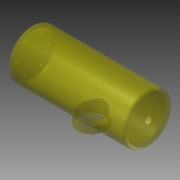
# Autodesk Inventor part: X-Ray Tube
Saved by Autodesk Inventor 2015 (Build 190159000, 159)
## iProperties
Created: 2015-03-02
Part Number: X-Ray Tube
Material: Glass
Document SubType Name: Modeling
Designer: pltwe4
Density: 2.18 g/cm^3
Appearance: Clear - Yellow
Author: pltwe4
Autodesk Inventor part; units mm, degrees
ref_plane "XZ Plane" through (0, 0, 0) normal (0, 1, 0) x (-1, 0, 0)
ref_plane "XY Plane" through (0, 0, 0) normal (0, 0, 1) x (1, 0, 0)
sketch "Sketch1" plane through (0, 0, 0) normal (0, 0, 1) x (1, 0, 0)
  circle A0 centre (0, 0) radius 14.925
  dimension "d0" = 29.85
  constraints: 1 centre point, 1 coincident
  measures "d0" diameter of A0
extrude "Extrusion1" add sketch "Sketch1" along normal mid plane 71.7
ref_plane "Work Plane1" through (14.925, 0, 0) normal (1, 0, 0) x (0, 1, 0)
sketch "Sketch2" plane through (14.925, 0, 0) normal (1, 0, 0) x (0, 1, 0)
  line L0 (-14.925, -35.85) -> (14.925, -35.85) projected
  line L1 (14.925, 35.85) -> (-14.925, 35.85) projected
  circle A0 centre (0, -1.03) radius 8.575
  line L2 (0, 50.19) -> (0, -50.19) projected
  circle A1 centre (0, -1.03) radius 7.575
  point P0 (0, 0)
  dimension "d3" = 34.82
  dimension "d4" = 17.15
  dimension "d49" = 1
  constraints: 2 centre point, 1 coincident, 1 point on line
  measures "d3" distance from line of L0 A0.centre
  measures "d4" diameter of A0
  measures "d49" radial gap between concentric circles of A1 A0
extrude "Extrusion2" add sketch "Sketch2" against normal up to surface round surface about axis through (0, 0, 0) along (0, 0, 1) radius 14.925 far side no
sketch "Sketch9" plane through (0, 0, 35.85) normal (0, 0, 1) x (1, 0, 0)
  point P0 (0, 0)
sketch "Sketch10" plane through (0, 0, 35.85) normal (0, 0, 1) x (1, 0, 0)
  circle A0 centre (0, 0) radius 12.925
  circle A1 centre (0, 0) radius 14.925 projected
  dimension "d31" = 2
  constraints: 1 centre point, 1 coincident
  measures "d31" radial gap between concentric circles of A1 A0
extrude "Extrusion11" cut sketch "Sketch10" against normal blind 70.7 contours A0
fillet "Fillet3" radius 2 1 edges at (-12.925, 0, -34.85)
fillet "Fillet4" radius 2 1 edges at (-14.925, 0, -35.85)
sketch "Sketch11" plane through (0, 0, 35.85) normal (0, 0, 1) x (1, 0, 0)
  circle A0 centre (0, 0) radius 12.925 projected
extrude "Extrusion12" add sketch "Sketch11" against normal blind 1
fillet "Fillet6" radius 2 1 edges at (-12.925, 0, 34.85)
fillet "Fillet7" radius 2 1 edges at (-14.925, 0, 35.85)
sketch "Sketch12" plane through (0, 0, -35.85) normal (0, 0, -1) x (-1, 0, 0)
  circle A0 centre (0, 0) radius 12.925 projected
  circle A1 centre (0, 0) radius 5.55
  circle A2 centre (0, 0) radius 2.032
  dimension "d42" = 11.1
  dimension "d43" = 4.064
  constraints: 2 centre point, 2 coincident
  measures "d42" diameter of A1
  measures "d43" diameter of A2
extrude "Extrusion13" cut sketch "Sketch12" against normal up to next contours A2
fillet "Fillet8" radius 2 5 edges at (13.6017, 6.1441, 4.9517) (12.2267, 8.5595, -0.514) (13.4268, 6.5174, -6.6026) (13.6009, -6.1459, 4.9499) (13.2583, -6.8537, -6.1833)
extrude "Extrusion15" cut sketch "Sketch2" against normal up to next contours A1 L2 | L2 A1
extrude "Extrusion16" add sketch "Sketch2" along normal blind 4 contours A0 L2 A1 | L2 A1 A0
sketch "Sketch13" plane through (0, 0, 35.85) normal (0, 0, 1) x (1, 0, 0)
  circle A0 centre (0, 0) radius 10 construction
  circle A1 centre (-8.6603, 5) radius 1.5
  circle A2 centre (-8.6603, 5) radius 0.75
  circle A3 centre (-8.6603, -5) radius 1.5
  circle A4 centre (-8.6603, -5) radius 0.75
  circle A5 centre (0, -10) radius 1.5
  circle A6 centre (0, -10) radius 0.75
  circle A7 centre (8.6603, -5) radius 1.5
  circle A8 centre (8.6603, -5) radius 0.75
  circle A9 centre (8.6603, 5) radius 1.5
  circle A10 centre (8.6603, 5) radius 0.75
  circle A11 centre (0, 10) radius 1.5
  circle A12 centre (0, 10) radius 0.75
  line L0 (-8.6603, -5) -> (-8.6603, 5) construction
  line L1 (0, 20.895) -> (0, -20.895) projected
  dimension "d54" = 20
  dimension "d55" = 3
  dimension "d56" = 1.5
  dimension "d59" = 360
  constraints: 12 centre point, 7 coincident, 2 end point, 1 parallel, 28 other
  measures "d55" diameter of A1
  measures "d56" diameter of A2
extrude "Extrusion17" cut sketch "Sketch13" against normal up to next contours A2 | A4 | L1 A6 | A6 L1 | A8 | A10 | L1 A12 | A12 L1
body "Solid1"
